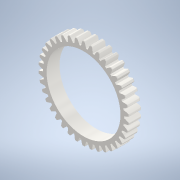
# Autodesk Inventor part: Цилиндрическое зубчатое зацепление1
Saved by Autodesk Inventor 2021 (Build 250183000, 183)
## iProperties
CustomPartVersion: 1
Created: 2021-03-23
Part Number: Цилиндрическое зубчатое зацепление1
Material: Steel
Document SubType Name: Modeling
Designer: Данил
Categories: <?xml version="1.0" encoding="UTF-16"?> <MemberInstance><Categories><FamilyTemplate><FamilyTemplateParameter ValueType="xs:double" Id="1" ObjectReferenceKey="da_z" ObjectType="kUserParameterObject"/><FamilyTemplateParameter ValueType="xs:double" Id="2" ObjectReferenceKey="da_b" ObjectType="kUserParameterObject"/><FamilyTemplateParameter ValueType="xs:double" Id="3" ObjectReferenceKey="da_beta" ObjectType="kUserParameterObject"/><FamilyTemplateParameter ValueType="xs:double" Id="4" ObjectReferenceKey="da_da" ObjectType="kUserParameterObject"/><FamilyTemplateParameter ValueType="xs:double" Id="5" ObjectReferenceKey="da_aw" ObjectType="kUserParameterObject"/><FamilyTemplateParameter ValueType="xs:string" Id="6" ObjectReferenceKey="EAIAABAAAACIAQAAAAAAAIAAAAAAAAAA" ObjectType="83910656" SubObjectId="SurfaceGeometry"/></FamilyTemplate><ParamToTemplateMap><ParamToTemplate CategoryParameter="//CategoryParameter[@InternalName='046C89C9-8512-4d59-83FE-43B91F4F132A']" TemplateParameter="1"/><ParamToTemplate CategoryParameter="//CategoryParameter[@InternalName='2552DF32-E462-4b46-AEBF-C6C7768E72AC']" TemplateParameter="2"/><ParamToTemplate CategoryParameter="//CategoryParameter[@InternalName='C9EE641D-15FC-4fae-A226-E94C4372FDD7']" TemplateParameter="3"/><ParamToTemplate><ParamToTemplate CategoryParameter="//CategoryParameter[@InternalName='00B6519A-459B-49c7-AD84-2E56D39A5744']" ConstantValue="-0.117500"/></ParamToTemplate><ParamToTemplate><ParamToTemplate CategoryParameter="//CategoryParameter[@InternalName='04B31F0E-C7A6-4894-AA32-9629BEFACF47']" ConstantValue="1.000000"/></ParamToTemplate><ParamToTemplate><ParamToTemplate CategoryParameter="//CategoryParameter[@InternalName='43CBEC2E-7847-49e7-A936-2F7889FCB2D9']" ConstantValue="0.250000"/></ParamToTemplate><ParamToTemplate><ParamToTemplate CategoryParameter="//CategoryParameter[@InternalName='B1EFC894-105D-4ebd-86BF-FA20ED196853']" ConstantValue="0.300000"/></ParamToTemplate><ParamToTemplate><ParamToTemplate CategoryParameter="//CategoryParameter[@InternalName='51175063-3D10-4879-93E8-6246FE8B403D']" ConstantValue="2060000000.000000"/></ParamToTemplate><ParamToTemplate><ParamToTemplate CategoryParameter="//CategoryParameter[@InternalName='A3A52E27-4454-46a9-B0BD-C932399B70AF']" ConstantValue="0.300000"/></ParamToTemplate><ParamToTemplate><ParamToTemplate CategoryParameter="//CategoryParameter[@InternalName='91B76062-C214-41d9-B1B9-14D2AB99603D']" ConstantValue="0.425000"/></ParamToTemplate><ParamToTemplate><ParamToTemplate CategoryParameter="//CategoryParameter[@InternalName='374E806E-8B8A-4dda-A9AA-1039D6500AD2']" ConstantValue="2.352941"/></ParamToTemplate><ParamToTemplate><ParamToTemplate CategoryParameter="//CategoryParameter[@InternalName='2D373A89-B862-43d6-8D0B-0CBF12AB9F6C']" ConstantValue="0.436332"/></ParamToTemplate><ParamToTemplate CategoryParameter="//CategoryParameter[@InternalName='37777632-D6A2-4fac-9D53-DB8ACD95C989']" TemplateParameter="4"/><ParamToTemplate CategoryParameter="//CategoryParameter[@InternalName='FD1017F1-B727-4f7e-9707-0F86F1FF9423']" TemplateParameter="5"/><ParamToTemplate><ParamToTemplate CategoryParameter="//CategoryParameter[@InternalName='9E1B4470-B2D3-4ff1-B813-535BB4CDF51A']" ConstantValue="3520000.000000"/></ParamToTemplate><ParamToTemplate><ParamToTemplate CategoryParameter="//CategoryParameter[@InternalName='F8452263-BFF6-458c-9FB1-07C4B99E95CD']" ConstantValue="11400000.000000"/></ParamToTemplate><ParamToTemplate><ParamToTemplate CategoryParameter="//CategoryParameter[@InternalName='3E3BB259-FD49-497f-8171-6EBC954A3479']" ConstantValue="2.000000"/></ParamToTemplate><ParamToTemplate CategoryParameter="//CategoryParameter[@InternalName='27C3BAF2-7550-4e4b-AE2C-0DB134B7D9B7']" TemplateParameter="6"/></ParamToTemplateMap><Category DisplayName="Gear" InternalName="DC85795E-93AB-48d5-8EEE-5A27447B64BD" Mnemonic="Gear"><CategoryParameter DisplayName="z" InternalName="046C89C9-8512-4d59-83FE-43B91F4F132A" Mnemonic="z"/><CategoryParameter DisplayName="b" InternalName="2552DF32-E462-4b46-AEBF-C6C7768E72AC" Mnemonic="b"/><CategoryParameter DisplayName="||b|" InternalName="C9EE641D-15FC-4fae-A226-E94C4372FDD7" Mnemonic="beta"/><CategoryParameter DisplayName="x" InternalName="00B6519A-459B-49c7-AD84-2E56D39A5744" Mnemonic="x"/><CategoryParameter DisplayName="a*" InternalName="04B31F0E-C7A6-4894-AA32-9629BEFACF47" Mnemonic="a"/><CategoryParameter DisplayName="c*" InternalName="43CBEC2E-7847-49e7-A936-2F7889FCB2D9" Mnemonic="c"/><CategoryParameter DisplayName="r|.f|*" InternalName="B1EFC894-105D-4ebd-86BF-FA20ED196853" Mnemonic="rf"/><CategoryParameter DisplayName="E" InternalName="51175063-3D10-4879-93E8-6246FE8B403D" Mnemonic="E"/><CategoryParameter DisplayName="||m|" InternalName="A3A52E27-4454-46a9-B0BD-C932399B70AF" Mnemonic="mi"/><Category DisplayName="SpurGear" InternalName="26C5A22E-A91E-4dfd-A3B3-23CCAFAE1764" Mnemonic="SpurGear"><CategoryParameter DisplayName="m" InternalName="91B76062-C214-41d9-B1B9-14D2AB99603D" Mnemonic="m"/><CategoryParameter DisplayName="P" InternalName="374E806E-8B8A-4dda-A9AA-1039D6500AD2" Mnemonic="PP"/><CategoryParameter DisplayName="||a|" InternalName="2D373A89-B862-43d6-8D0B-0CBF12AB9F6C" Mnemonic="alpha"/><CategoryParameter DisplayName="d|.a|" InternalName="37777632-D6A2-4fac-9D53-DB8ACD95C989" Mnemonic="da"/><CategoryParameter DisplayName="a|.w|" InternalName="FD1017F1-B727-4f7e-9707-0F86F1FF9423" Mnemonic="aw"/><CategoryParameter DisplayName="||s||.Flim|" InternalName="9E1B4470-B2D3-4ff1-B813-535BB4CDF51A" Mnemonic="sFlim"/><CategoryParameter DisplayName="||s||.Hlim|" InternalName="F8452263-BFF6-458c-9FB1-07C4B99E95CD" Mnemonic="sHlim"/><CategoryParameter DisplayName="тип" InternalName="3E3BB259-FD49-497f-8171-6EBC954A3479" Mnemonic="type"/><CategoryParameter DisplayName="PitchDiameter" InternalName="27C3BAF2-7550-4e4b-AE2C-0DB134B7D9B7" Mnemonic="IDS_PITCHDIAM"/></Category></Category></Categories></MemberInstance>
Density: 1 g/cm^3
Appearance: Steel
Author: Данил
Autodesk Inventor part; units mm, degrees
sketch "Sketch1" plane through (0, 0, 0) normal (0, 0, 1) x (1, 0, 0)
  circle A0 centre (0, 0) radius 84.5006
  dimension "d0" = 169.0012
  constraints: 1 centre point
  measures "d0" diameter of A0
extrude "Extrusion1" add sketch "Sketch1" along normal blind 24
ref_plane "Work Plane2" through (0, 0, 12) normal (0, 0, 1) x (1, 0, 0)
sketch "Sketch2" plane through (0, 0, 0) normal (0, 0, -1) x (-1, 0, 0)
  circle A0 centre (0, 0) radius 84.5006 projected
  circle A1 centre (0, 0) radius 80.75
  dimension "d3" = 161.5
  constraints: 1 centre point, 1 coincident
  measures "d3" diameter of A1
surface extrude "Средний диаметр" sketch "Sketch2" against normal through all shown no curves A1
ref_plane "Work Plane8" through (0, 0, 0) normal (0.9965845, 0.0825793, 0) x (0, 0, 1)
ref_plane "Work Plane9" through (0, 0, 0) normal (1, 0, 0) x (0, 1, 0)
spur gear teeth "Цилиндрическое зубчатое зацепление" teeth 38 pitch diameter 161.5 tip diameter 169.0012 root diameter 149.8763 face width 24 start plane through (0, 0, 0) normal (0, 0, -1) x (-1, 0, 0)
sketch "Эскиз3" plane through (0, 0, 24) normal (0, 0, 1) x (1, 0, 0)
  circle A0 centre (0, 0) radius 68.5
  dimension "d49" = 137
  constraints: 1 centre point, 1 coincident
  measures "d49" diameter of A0
extrude "Выдавливание2" cut sketch "Эскиз3" against normal through all
chamfer "Фаска1" distance 1.8 angle 45 38 edges at (77.3834, -33.9435, 0) (81.9149, -20.7437, 0) (84.212, -6.978, 0) (84.212, 6.978, 0) (81.9149, 20.7437, 0) (77.3834, 33.9435, 0) (70.7411, 46.2175, 0) (62.1691, 57.2307, 0) (51.9014, 66.6829, 0) (40.2179, 74.3161, 0) (27.4373, 79.9221, 0) (13.9083, 83.3481, 0) (0, 84.5006, 0) (-13.9083, 83.3481, 0) (-27.4373, 79.9221, 0) (-40.2179, 74.3161, 0) (-51.9014, 66.6829, 0) (-62.1691, 57.2307, 0) (-70.7411, 46.2175, 0) (-77.3834, 33.9435, 0) (-81.9149, 20.7437, 0) (-84.212, 6.978, 0) (-84.212, -6.978, 0) (-81.9149, -20.7437, 0) (-77.3834, -33.9435, 0) (-70.7411, -46.2175, 0) (-62.1691, -57.2307, 0) (-51.9014, -66.6829, 0) (-40.2179, -74.3161, 0) (-27.4373, -79.9221, 0) (-13.9083, -83.3481, 0) (0, -84.5006, 0) (13.9083, -83.3481, 0) (27.4373, -79.9221, 0) (40.2179, -74.3161, 0) (51.9014, -66.6829, 0) (62.1691, -57.2307, 0) (70.7411, -46.2175, 0)
chamfer "Фаска2" distance 0.8 angle 45 38 edges at (84.212, -6.978, 24) (81.9149, -20.7437, 24) (77.3834, -33.9435, 24) (70.7411, -46.2175, 24) (62.1691, -57.2307, 24) (51.9014, -66.6829, 24) (40.2179, -74.3161, 24) (27.4373, -79.9221, 24) (13.9083, -83.3481, 24) (0, -84.5006, 24) (-13.9083, -83.3481, 24) (-27.4373, -79.9221, 24) (-40.2179, -74.3161, 24) (-51.9014, -66.6829, 24) (-62.1691, -57.2307, 24) (-70.7411, -46.2175, 24) (-77.3834, -33.9435, 24) (-81.9149, -20.7437, 24) (-84.212, -6.978, 24) (-84.212, 6.978, 24) (-81.9149, 20.7437, 24) (-77.3834, 33.9435, 24) (-70.7411, 46.2175, 24) (-62.1691, 57.2307, 24) (-51.9014, 66.6829, 24) (-40.2179, 74.3161, 24) (-27.4373, 79.9221, 24) (-13.9083, 83.3481, 24) (0, 84.5006, 24) (13.9083, 83.3481, 24) (27.4373, 79.9221, 24) (40.2179, 74.3161, 24) (51.9014, 66.6829, 24) (62.1691, 57.2307, 24) (70.7411, 46.2175, 24) (77.3834, 33.9435, 24) (81.9149, 20.7437, 24) (84.212, 6.978, 24)
chamfer "Фаска3" distance 0.3 angle 45 2 edges at (81.4687, -22.4322, 12.5) (82.3261, -19.0463, 12.5)
chamfer "Фаска4" distance 0.3 angle 45 2 edges at (84.0498, -8.7169, 12.5) (84.3382, -5.2361, 12.5)
chamfer "Фаска5" distance 0.3 angle 45 2 edges at (84.3382, 5.2361, 12.5) (84.0498, 8.7169, 12.5)
chamfer "Фаска6" distance 0.3 angle 45 20 edges at (82.3261, 19.0463, 12.5) (81.4687, 22.4322, 12.5) (78.0684, 32.337, 12.5) (76.6654, 35.5355, 12.5) (71.6812, 44.7456, 12.5) (69.7708, 47.6696, 12.5) (63.3386, 55.9336, 12.5) (60.9731, 58.5033, 12.5) (53.2684, 65.596, 12.5) (50.5121, 67.7413, 12.5) (41.7451, 73.469, 12.5) (38.6734, 75.1314, 12.5) (29.0832, 79.338, 12.5) (25.7797, 80.4721, 12.5) (15.6279, 83.0429, 12.5) (12.1828, 83.6178, 12.5) (1.7464, 84.4826, 12.5) (-1.7464, 84.4826, 12.5) (-12.1828, 83.6178, 12.5) (-15.6279, 83.0429, 12.5)
chamfer "Фаска7" distance 0.3 angle 45 6 edges at (-25.7797, 80.4721, 12.5) (-29.0832, 79.338, 12.5) (-38.6734, 75.1314, 12.5) (-41.7451, 73.469, 12.5) (-50.5121, 67.7413, 12.5) (-53.2684, 65.596, 12.5)
chamfer "Фаска8" distance 0.3 angle 45 12 edges at (-60.9731, 58.5033, 12.5) (-63.3386, 55.9336, 12.5) (-69.7708, 47.6696, 12.5) (-71.6812, 44.7456, 12.5) (-76.6654, 35.5355, 12.5) (-78.0684, 32.337, 12.5) (-81.4687, 22.4322, 12.5) (-82.3261, 19.0463, 12.5) (-84.0498, 8.7169, 12.5) (-84.3382, 5.2361, 12.5) (-84.3382, -5.2361, 12.5) (-84.0498, -8.7169, 12.5)
chamfer "Фаска9" distance 0.3 angle 45 26 edges at (-82.3261, -19.0463, 12.5) (-81.4687, -22.4322, 12.5) (-78.0684, -32.337, 12.5) (-76.6654, -35.5355, 12.5) (-71.6812, -44.7456, 12.5) (-69.7708, -47.6696, 12.5) (-63.3386, -55.9336, 12.5) (-60.9731, -58.5033, 12.5) (-53.2684, -65.596, 12.5) (-50.5121, -67.7413, 12.5) (-41.7451, -73.469, 12.5) (-38.6734, -75.1314, 12.5) (-29.0832, -79.338, 12.5) (-25.7797, -80.4721, 12.5) (-15.6279, -83.0429, 12.5) (-12.1828, -83.6178, 12.5) (-1.7464, -84.4826, 12.5) (1.7464, -84.4826, 12.5) (12.1828, -83.6178, 12.5) (15.6279, -83.0429, 12.5) (25.7797, -80.4721, 12.5) (29.0832, -79.338, 12.5) (38.6734, -75.1314, 12.5) (41.7451, -73.469, 12.5) (50.5121, -67.7413, 12.5) (53.2684, -65.596, 12.5)
chamfer "Фаска10" distance 0.3 angle 45 6 edges at (60.9731, -58.5033, 12.5) (63.3386, -55.9336, 12.5) (69.7708, -47.6696, 12.5) (71.6812, -44.7456, 12.5) (76.6654, -35.5355, 12.5) (78.0684, -32.337, 12.5)
equation "\"d0\" = da_da"
equation "\"d1\" = da_b"
equation "\"d3\" = da_d"
equation "\"d16\" = da_aw"
equation "\"d43\" = da_aw"
equation "\"d46\" = da_aw"
equation "\"da_da\" = 169.00125"
equation "\"da_b\" = 24"
equation "\"da_d\" = 161.5"
equation "\"da_aw\" = 233.75"
body "Solid1"
body "Srf1"
